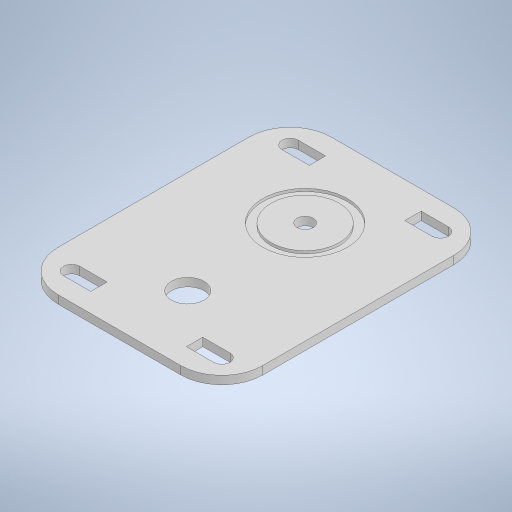
# Autodesk Inventor part: Plate
Saved by Autodesk Inventor 2024.1 (Build 281209000, 209)
## iProperties
Created: 2023-12-30
Part Number: Plate
Material: Generic
Document SubType Name: Modeling
Designer: ryanm
Density: 1 g/cm^3
Appearance: Default
Author: ryanm
Autodesk Inventor part; units mm, degrees
ref_plane "YZ Plane" through (0, 0, 0) normal (1, 0, 0) x (0, 1, 0)
ref_plane "XZ Plane" through (0, 0, 0) normal (0, 1, 0) x (-1, 0, 0)
ref_plane "XY Plane" through (0, 0, 0) normal (0, 0, 1) x (1, 0, 0)
sketch "Sketch1" plane through (0, 0, 0) normal (0, 1, 0) x (-1, 0, 0)
  line L0 (37.5, -50) -> (-37.5, -50)
  line L1 (-37.5, -50) -> (-37.5, 50)
  line L2 (-37.5, 50) -> (37.5, 50)
  line L3 (37.5, 50) -> (37.5, -50)
  point P0 (0, 0)
  point P1 (0, -50)
  point P2 (37.5, 0)
  dimension "d0" = 75
  dimension "d1" = 100
  constraints: 8 end point, 2 midpoint, 2 parallel, 1 horizontal, 1 horizontal alignment, 1 perpendicular, 1 vertical alignment
  measures "d0" distance of L0.start L0.end
  measures "d1" distance of L2.end L0.start
extrude "Extrusion1" add sketch "Sketch1" along normal blind 3
sketch "Sketch2" plane through (0, 3, 0) normal (0, 1, 0) x (1, 0, 0)
  arc A0 (-27.5, 43) -> (-27.5, 37) centre (-27.5, 40) ccw
  arc A1 (27.5, 37) -> (27.5, 43) centre (27.5, 40) ccw
  arc A2 (27.5, -43) -> (27.5, -37) centre (27.5, -40) ccw
  arc A3 (-27.5, -37) -> (-27.5, -43) centre (-27.5, -40) ccw
  line L0 (37.5, 50) -> (-37.5, 50) projected
  line L1 (-37.5, 50) -> (-37.5, -50) projected
  line L2 (-37.5, -50) -> (37.5, -50) projected
  line L3 (37.5, -50) -> (37.5, 50) projected
  line L4 (-27.5, -37) -> (-17.5, -37)
  line L5 (-17.5, -37) -> (-17.5, -43)
  line L6 (-17.5, -43) -> (-27.5, -43)
  line L7 (27.5, -37) -> (17.5, -37)
  line L8 (27.5, -43) -> (17.5, -43)
  line L9 (17.5, -37) -> (17.5, -43)
  line L10 (-27.5, 43) -> (-17.5, 43)
  line L11 (-17.5, 43) -> (-17.5, 37)
  line L12 (-17.5, 37) -> (-27.5, 37)
  line L13 (27.5, 43) -> (17.5, 43)
  line L14 (17.5, 43) -> (17.5, 37)
  line L15 (17.5, 37) -> (27.5, 37)
  point P0 (0, 0)
  dimension "d4" = 6
  dimension "d5" = 6
  dimension "d6" = 6
  dimension "d7" = 6
  dimension "d8" = 10
  dimension "d9" = 10
  dimension "d10" = 10
  dimension "d11" = 10
  dimension "d29" = 6
  dimension "d32" = 10
  dimension "d34" = 6
  dimension "d35" = 10
  dimension "d36" = 6
  dimension "d37" = 10
  dimension "d38" = 10
  dimension "d39" = 6
  constraints: 24 end point, 8 point on circle, 6 tangent, 5 horizontal, 4 centre point, 3 perpendicular, 2 horizontal alignment, 2 vertical alignment, 1 vertical
  measures "d4" diameter of A0
  measures "d5" diameter of A1
  measures "d6" diameter of A3
  measures "d7" diameter of A2
  measures "d8" distance from line of L0 A0.centre
  measures "d9" distance from line of L1 A0.centre
  measures "d10" distance from line of L2 A2.centre
  measures "d11" distance from line of L3 A2.centre
  measures "d29" distance between parallel lines of L6 L4
  measures "d32" distance of L5.end L6.end
  measures "d34" distance between parallel lines of L8 L7
  measures "d35" distance from line of A2.centre L9
  measures "d36" distance of L10.end L11.end
  measures "d37" distance from line of L11 L12.end
  measures "d38" distance from line of L15.end L14
  measures "d39" distance of L13.end L14.end
extrude "Extrusion2" cut sketch "Sketch2" against normal blind 3 contours L10 L11 L12 A0 | L15 L14 L13 A1 | L8 L9 L7 A2 | L4 L5 L6 A3
sketch "Sketch3" plane through (0, 3, 0) normal (0, 1, 0) x (1, 0, 0)
  circle A0 centre (0, -25) radius 6
  point P0 (0, 0)
  dimension "d17" = 12
  dimension "d18" = 25
  constraints: 1 centre point, 1 vertical alignment
  measures "d17" diameter of A0
  measures "d18" distance of A0.centre point (0, 0)
extrude "Extrusion3" cut sketch "Sketch3" against normal through all
sketch "Sketch4" plane through (0, 3, 0) normal (0, 1, 0) x (1, 0, 0)
  circle A0 centre (0, 18) radius 15.5
  circle A1 centre (0, 18) radius 12.5
  point P0 (0, 0)
  dimension "d20" = 3
  dimension "d21" = 18
  dimension "d28" = 25
  constraints: 2 centre point, 1 vertical alignment
  measures "d20" radial gap between concentric circles of A0 A1
  measures "d21" distance of point (0, 0) A0.centre
  measures "d28" diameter of A1
extrude "Extrusion4" cut sketch "Sketch4" against normal blind 1
sketch "Sketch5" plane through (0, 3, -18) normal (0, 1, 0) x (1, 0, 0)
  circle A0 centre (0, 0) radius 3
  circle A1 centre (0, 0) radius 12.5 projected
  point P0 (0, -18)
  dimension "d24" = 6
  constraints: 1 centre point, 1 concentric, 1 vertical alignment
  measures "d24" diameter of A0
extrude "Extrusion5" cut sketch "Sketch5" against normal through all contours A0
fillet "Fillet1" radius 15 4 edges at (-37.5, 1.5, 50) (37.5, 1.5, 50) (37.5, 1.5, -50) (-37.5, 1.5, -50)
equation "\"d5\" = d4"
equation "\"d6\" = d4"
equation "\"d7\" = d4"
equation "\"d9\" = d8"
equation "\"d10\" = d8"
equation "\"d11\" = d9"
equation "\"d29\" = d6"
equation "\"d34\" = d7"
equation "\"d35\" = d32"
equation "\"d36\" = d4"
equation "\"d37\" = d32"
equation "\"d38\" = d37"
equation "\"d39\" = d5"
body "Solid1"
